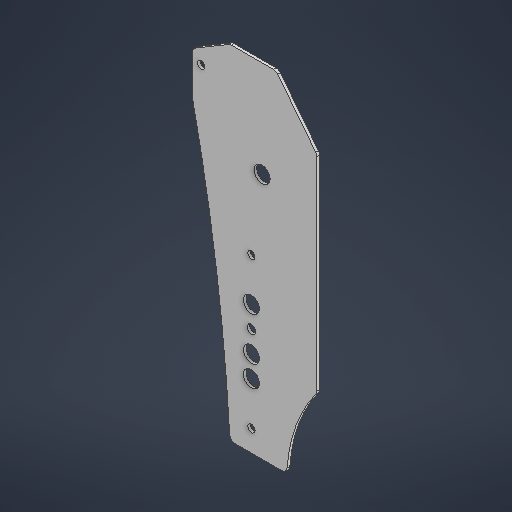
# Autodesk Inventor part: Part3
Saved by Autodesk Inventor 2026.1 (Build 301233000, 233)
## iProperties
Created: 2026-03-06
Part Number: Part3
Material: Generic
Document SubType Name: Modeling
Designer: roejo
Density: 1 g/cm^3
Appearance: Default
Author: roejo
Autodesk Inventor part; units mm, degrees
ref_plane "YZ Plane" through (0, 0, 0) normal (1, 0, 0) x (0, 1, 0)
ref_plane "XZ Plane" through (0, 0, 0) normal (0, 1, 0) x (-1, 0, 0)
ref_plane "XY Plane" through (0, 0, 0) normal (0, 0, 1) x (1, 0, 0)
sketch "Sketch1" plane through (0, 0, 0) normal (0, 0, 1) x (1, 0, 0)
  line L0 (377.0029, 160.9063) -> (356.3654, 160.9063)
  circle A0 centre (336.9408, 141.8563) radius 2.1844
  line L1 (331.7592, 123.8223) -> (331.7592, 147.1903)
  line L2 (331.7592, 147.1903) -> (332.7752, 148.2063)
  line L3 (332.7752, 148.2063) -> (342.0779, 148.2063)
  line L4 (356.3654, 160.9063) -> (353.9842, 160.9063)
  line L5 (354.8564, 160.9063) -> (379.7418, 160.9063)
  line L6 (382.24, 159.6907) -> (404.7811, 130.9525)
  line L7 (405.4579, 128.993) -> (405.4579, 8.9191)
  line L8 (353.2344, 160.4607) -> (333.3122, 148.6212)
  line L9 (331.7592, 145.8918) -> (331.7592, 122.4835)
  arc A1 (404.8445, 7.0432) -> (387.8405, -39.3429) centre (476.7839, -45.6377) ccw
  line L10 (384.6734, -42.2937) -> (356.983, -42.2937)
  arc A2 (353.8134, -39.3043) -> (331.7592, 122.4835) centre (-705.6943, -101.3347) ccw
  arc A3 (333.3122, 148.6212) -> (331.7592, 145.8918) centre (334.9342, 145.8918) ccw
  arc A4 (354.8564, 160.9063) -> (353.2344, 160.4607) centre (354.8564, 157.7313) ccw
  arc A5 (382.24, 159.6907) -> (379.7418, 160.9063) centre (379.7418, 157.7313) ccw
  arc A6 (405.4579, 128.993) -> (404.7811, 130.9525) centre (402.2829, 128.993) ccw
  arc A7 (404.8445, 7.0432) -> (405.4579, 8.9191) centre (402.2829, 8.9191) ccw
  arc A8 (384.6734, -42.2937) -> (387.8405, -39.3429) centre (384.6734, -39.1187) ccw
  arc A9 (353.8134, -39.3043) -> (356.983, -42.2937) centre (356.983, -39.1187) ccw
  circle A10 centre (373.0342, 103.7563) radius 4.7625
  circle A11 centre (366.6842, 59.3063) radius 2.1844
  circle A12 centre (366.6842, 21.2063) radius 2.54
  circle A13 centre (366.6842, 33.9063) radius 4.7625
  circle A14 centre (366.6842, 8.5063) radius 4.7625
  circle A15 centre (366.6842, -4.1937) radius 4.7625
  circle A16 centre (366.6842, -29.5937) radius 2.1844
  point P0 (0, 0)
  point P1 (405.4579, 7.8708)
  point P2 (387.6807, -42.2937)
  point P3 (353.9842, -42.2937)
  dimension "d1" = 3.175
  dimension "d2" = 3.175
  dimension "d3" = 9.525
  dimension "d4" = 4.3688
  dimension "d5" = 5.08
  dimension "d6" = 9.525
  dimension "d7" = 9.525
  dimension "d8" = 9.525
  dimension "d9" = 4.3688
  constraints: 22 end point, 21 point on circle, 17 centre point, 14 tangent, 6 point on line, 5 equal radius, 2 horizontal, 1 perpendicular
  measures "d1" radius of A3
  measures "d2" radius of A4
  measures "d3" diameter of A10
  measures "d4" diameter of A11
  measures "d5" diameter of A12
  measures "d6" diameter of A13
  measures "d7" diameter of A14
  measures "d8" diameter of A15
  measures "d9" diameter of A16
extrude "Extrusion1" add sketch "Sketch1" along normal blind 1.5875 contours L5 A5 L6 A6 L7 A7 A1 A8 L10 A9 A2 L9 L1 A3 L8 A4 L4 L0
body "Solid1"
